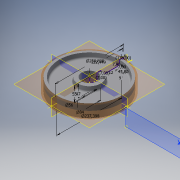
# Autodesk Inventor part: Колесл тихоходное
Saved by Autodesk Inventor 2018 (Build 220112000, 112)
## iProperties
Created: 2018-03-25
Part Number: Колесл тихоходное
Material: Типовые
Document SubType Name: Modeling
Designer: kriku
Density: 1 g/cm^3
Appearance: По умолчанию
Author: kriku
Autodesk Inventor part; units mm, degrees
sketch "Эскиз1" plane through (0, 0, 0) normal (1, 0, 0) x (0, 1, 0)
  line L0 (0, 23.5) -> (0, -23.5)
  line L1 (125.449, 0) -> (-30.3457, 0)
  line L2 (28, 23.5) -> (28, -31.5)
  line L3 (28, -31.5) -> (42, -31.5)
  line L4 (42, -31.5) -> (42, -6)
  line L5 (50.4394, -6) -> (102.2419, -6)
  line L6 (109.699, -6) -> (109.699, -23.5)
  line L7 (109.699, -23.5) -> (118.699, -23.5)
  line L8 (118.699, -23.5) -> (118.699, 23.5)
  line L9 (118.699, 23.5) -> (109.699, 23.5)
  line L10 (109.699, 23.5) -> (109.699, 6)
  line L11 (102.2419, 6) -> (49.4571, 6)
  line L12 (42, 6) -> (42, 23.5)
  line L13 (28, 23.5) -> (42, 23.5)
  line L14 (122.449, 7.3449) -> (122.449, -39.6551)
  line L15 (125.449, 21.9) -> (125.449, -21.9)
  line L16 (123.849, 23.5) -> (118.699, 23.5)
  line L17 (123.849, -23.5) -> (118.699, -23.5)
  line L18 (109.699, 23.5) -> (108.1972, 11.2688)
  line L19 (109.699, -23.5) -> (108.1972, -11.2688)
  line L20 (42, -31.5) -> (44.4841, -11.2688)
  line L21 (42, 23.5) -> (43.5018, 11.2688)
  arc A0 (102.2419, 6) -> (108.1972, 11.2688) centre (102.2419, 12) ccw
  arc A1 (108.1972, -11.2688) -> (102.2419, -6) centre (102.2419, -12) ccw
  arc A2 (50.4394, -6) -> (44.4841, -11.2688) centre (50.4394, -12) ccw
  arc A3 (43.5018, 11.2688) -> (49.4571, 6) centre (49.4571, 12) ccw
  line L22 (125.449, 21.9) -> (123.849, 23.5)
  line L23 (125.449, -21.9) -> (123.849, -23.5)
  line L24 (-61.5046, 0) -> (156.6079, 0) projected
  line L25 (0, -52.2861) -> (0, 36.131) projected
  point P0 (0, 0)
  point P1 (114.199, 23.5)
  point P2 (35, 23.5)
  point P3 (114.199, -23.5)
  dimension "d0" = 47
  dimension "d1" = 12
  dimension "d2" = 9
  dimension "d3" = 56
  dimension "d4" = 55
  dimension "d5" = 84
  dimension "d6" = 237.398
  dimension "d7" = 122.449
  dimension "d8" = 250.898
  dimension "d9" = 7
  dimension "d10" = 7
  dimension "d11" = 7
  dimension "d12" = 7
  dimension "d13" = 6
  dimension "d14" = 135
  dimension "d15" = 135
  dimension "d16" = 1.6
  dimension "d17" = 1.6
  constraints: 48 end point, 11 perpendicular, 10 point on line, 8 point on circle, 8 tangent, 5 parallel, 4 centre point, 4 midpoint, 4 vertical, 3 equal radius, 3 horizontal alignment, 2 symmetric about line, 1 collinear, 1 horizontal, 3 other
  measures "d0" distance of L0.start L0.end
  measures "d1" distance between parallel lines of L5 L11
  measures "d2" distance between parallel lines of L6 L8
  measures "d3" diameter of L2 L0
  measures "d4" distance of L2.start L2.end
  measures "d5" diameter of L4 L0
  measures "d6" diameter of L8 L0
  measures "d7" distance between parallel lines of L0 L14
  measures "d8" diameter of L15 L0
  measures "d9" angle of L10 L18
  measures "d10" angle of L19 L6
  measures "d11" angle of L12 L21
  measures "d12" angle of L4 L20
  measures "d13" radius of A0
  measures "d14" angle of L15 L23
  measures "d15" angle of L22 L15
  measures "d16" horizontal distance of L16.start L15.start
  measures "d17" horizontal distance of L17.start L15.end
revolve "Вращение1" add sketch "Эскиз1" angle 360 about axis through (0, 0, 23.5) along (0, 0, -1) contours L8 L7 L19 A1 L5 A2 L20 L3 L2 L1 | L1 L2 L13 L21 A3 L11 A0 L18 L9 L8
surface revolve "ВращПврх1" sketch "Эскиз1" angle 360 about axis through (0, 0, 23.5) along (0, 0, -1) shown yes curves L16 L22 L15 L23 L17
body "SRF1"
